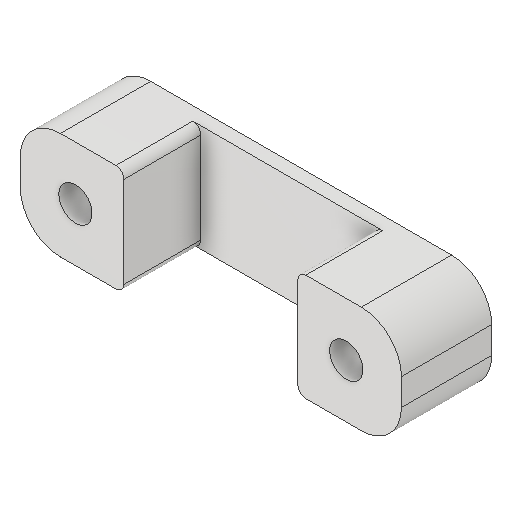
# Autodesk Inventor part: 3DP_PLA_X_axis_endstop_mount
Saved by Autodesk Inventor 2025 (Build 290162010, 162A)
## iProperties
Created: 2018-08-01
Part Number: 3DP_PLA_X_axis_endstop_mount
Material: ABS Plastic
Document SubType Name: Modeling
Designer: Andrzej
Density: 1.06 g/cm^3
Appearance: Smooth - White
Author: Andrzej
Autodesk Inventor part; units mm, degrees
ref_plane "YZ Plane" through (0, 0, 0) normal (1, 0, 0) x (0, 1, 0)
ref_plane "XZ Plane" through (0, 0, 0) normal (0, 1, 0) x (-1, 0, 0)
ref_plane "XY Plane" through (0, 0, 0) normal (0, 0, 1) x (1, 0, 0)
sketch "Sketch1" plane through (0, 0, 0) normal (0, 0, 1) x (1, 0, 0)
  line L0 (-3.0875, 5.2222) -> (9.9125, 5.2222)
  line L1 (9.9125, 5.2222) -> (9.9125, -2.7778)
  line L2 (9.9125, -2.7778) -> (-3.0875, -2.7778)
  line L3 (-3.0875, -2.7778) -> (-3.0875, 5.2222)
  line L4 (-3.0875, 5.2222) -> (-10.8375, 5.2222)
  line L5 (-10.8375, 5.2222) -> (-10.8375, -2.7778)
  line L6 (-10.8375, -2.7778) -> (-3.0875, -2.7778)
  line L7 (9.9125, -2.7778) -> (17.6625, -2.7778)
  line L8 (17.6625, -2.7778) -> (17.6625, 5.2222)
  line L9 (17.6625, 5.2222) -> (9.9125, 5.2222)
  point P0 (0, 0)
  point P1 (-6.7125, 1.2222)
  point P2 (13.5375, 1.2222)
  dimension "d0" = 13
  dimension "d1" = 8
  dimension "d2" = 7.75
  dimension "d3" = 7.75
  dimension "d6" = 4
  dimension "d7" = 4
  dimension "d22" = 20.25
  dimension "d23" = 28.5
  dimension "d24" = 4.125
  constraints: 20 end point, 5 perpendicular, 2 horizontal, 2 parallel, 2 point on line
  measures "d0" distance of L1.end L2.end
  measures "d1" distance of L2.end L0.start
  measures "d2" distance between parallel lines of L5 L3
  measures "d3" distance between parallel lines of L8 L1
  measures "d6" distance from line of L6 point (-6.713, 1.222)
  measures "d7" distance from line of L7 point (13.537, 1.222)
  measures "d22" distance of point (-6.713, 1.222) point (13.537, 1.222)
  measures "d23" distance between parallel lines of L5 L8
  measures "d24" distance from line of L5 point (-6.713, 1.222)
extrude "Extrusion1" add sketch "Sketch1" along normal blind 5.75 contours L3 L6 L5 L4 | L9 L8 L7 L1
extrude "Extrusion2" add sketch "Sketch1" against normal blind 1
hole "Hole1" at (-6.7125, 1.2222, 0) at (13.5375, 1.2222, 0) direction (0, 0, 1) diameter 2.5 end through all both
fillet "Fillet1" radius 3 4 edges at (-10.8375, -2.7778, 2.375) (-10.8375, 5.2222, 2.375) (17.6625, -2.7778, 2.375) (17.6625, 5.2222, 2.375)
fillet "Fillet2" radius 0.6 4 edges at (9.9125, -2.7778, 2.875) (-3.0875, -2.7778, 2.875) (9.9125, 5.2222, 2.875) (-3.0875, 5.2222, 2.875)
equation "\"d3\" = d2"
equation "\"d6\" = 0.5 * d1"
equation "\"d7\" = d6"
equation "\"d24\" = -0.5 * d22 + 0.5 * d23"
body "Solid1"
